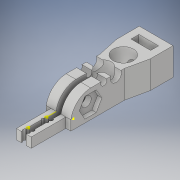
# Autodesk Inventor part: NeuroprobeholdermajigerV3.5SmallerstillStrongerNut
Saved by Autodesk Inventor 2017 (Build 210142000, 142)
## iProperties
Created: 2016-09-01
Part Number: NeuroprobeholdermajigerV3.5SmallerstillStrongerNut
Material: Generic
Document SubType Name: Modeling
Designer: andrew
Density: 1 g/cm^3
Appearance: Default
Author: andrew
Autodesk Inventor part; units mm, degrees
ref_plane "YZ Plane" through (0, 0, 0) normal (1, 0, 0) x (0, 1, 0)
ref_plane "XZ Plane" through (0, 0, 0) normal (0, 1, 0) x (-1, 0, 0)
ref_plane "XY Plane" through (0, 0, 0) normal (0, 0, 1) x (1, 0, 0)
sketch "Sketch1" plane through (0, 0, 0) normal (0, 1, 0) x (-1, 0, 0)
  line L0 (10.16, 7.62) -> (10.16, -36.068)
  line L1 (0, -36.068) -> (0, 3.81) construction
  circle A0 centre (5.08, -25.908) radius 2.9655
  line L2 (10.16, 7.62) -> (6.096, 7.62) construction
  line L3 (3.9775, 7.62) -> (0.0978, 7.62) construction
  line L4 (4.064, 3.81) -> (4.064, -11.0001) construction
  arc A1 (4.064, -14.8101) -> (6.096, -14.812) centre (5.0772, -17.8191) ccw
  line L5 (5.08, -31.75) -> (24.746, -31.75) construction
  line L6 (0, -4.7834) -> (2.794, -4.7834) construction
  line L7 (2.794, -13.6734) -> (0, -13.6734) construction
  line L8 (0, -13.6734) -> (0, -4.7834) construction
  line L9 (4.064, -4.7834) -> (0, -4.7834) construction
  line L10 (5.08, -31.75) -> (9.398, -31.75) construction
  line L11 (10.16, 7.62) -> (6.096, 7.62)
  line L12 (4.064, 7.62) -> (0, 7.62)
  line L13 (0, 0) -> (0, -36.068)
  line L14 (5.08, -36.068) -> (8.255, -36.068) construction
  line L15 (10.16, -36.068) -> (10.16, -39.243)
  line L16 (10.16, -39.243) -> (0, -39.243)
  line L17 (0, -39.243) -> (0, -36.068)
  line L18 (5.0772, -17.8191) -> (26.8769, -17.8191) construction
  arc A2 (4.064, 7.0772) -> (4.064, 5.9038) centre (4.307, 6.4905) ccw
  line L19 (4.064, 7.0772) -> (4.064, 7.62)
  arc A3 (4.064, 5.6778) -> (4.064, 4.0999) centre (4.307, 4.8889) ccw
  line L20 (4.064, -7.1901) -> (4.064, 4.0999)
  line L21 (4.064, 5.6778) -> (4.064, 5.9038)
  line L22 (4.064, 4.0999) -> (4.064, 3.81) construction
  line L23 (4.064, 7.62) -> (4.064, 7.0772) construction
  line L24 (4.064, 5.9038) -> (4.064, 5.6778) construction
  arc A4 (6.0904, 5.9038) -> (6.0904, 7.0772) centre (5.8475, 6.4905) ccw
  arc A5 (6.0904, 4.0999) -> (6.0904, 5.6778) centre (5.8475, 4.8889) ccw
  line L25 (6.096, 7.0749) -> (6.096, 7.62) construction
  line L26 (6.096, 4.1017) -> (6.096, -14.812)
  line L27 (6.096, 7.62) -> (6.096, 7.0749)
  line L28 (6.096, 5.9062) -> (6.096, 5.6761)
  line L29 (6.096, 3.81) -> (6.096, 4.1017) construction
  line L30 (6.096, 5.6761) -> (6.096, 5.9062) construction
  line L31 (0, 0) -> (0, 7.62)
  line L32 (4.064, -7.1901) -> (4.064, -14.8101)
  dimension "d0" = 10.16
  dimension "d1" = 5.9309
  dimension "d2" = 33.528
  dimension "d3" = 6.35
  constraints: 66 end point, 14 point on circle, 10 perpendicular, 6 centre point, 6 horizontal, 4 point on line, 4 vertical, 2 parallel, 1 collinear
  measures "d0" distance of L0.end L1.start
  measures "d1" diameter of A0
  measures "d2" distance from line of L2 A0.centre
  measures "d3" diameter of A1
extrude "Extrusion1" add sketch "Sketch1" along normal blind 4.064
sketch "Sketch3" plane through (0, 0, 7.62) normal (1, 0, 0) x (0, 0, -1)
  line L0 (3.5183, 0) -> (14.9483, 0) construction
  line L1 (3.5183, 0) -> (14.9483, 0) construction
  line L2 (14.9483, 0) -> (14.9483, 3.81) construction
  line L3 (19.5929, 8.2094) -> (17.2434, 4.14) construction
  line L4 (17.2434, 4.14) -> (12.5444, 4.14) construction
  line L5 (12.5444, 4.14) -> (10.1949, 8.2094) construction
  line L6 (10.1949, 8.2094) -> (12.5444, 12.2789) construction
  line L7 (12.5444, 12.2789) -> (17.2434, 12.2789) construction
  line L8 (17.2434, 12.2789) -> (19.5929, 8.2094) construction
  line L9 (14.8939, 4.14) -> (14.8939, 5.4124) construction
  line L10 (10.1949, 8.2094) -> (6.3849, 8.2094) construction
  line L11 (22.4301, 4.064) -> (3.5201, 4.064) construction
  line L12 (10.1949, 8.2094) -> (14.0049, 8.2094) construction
  line L13 (6.3849, 8.2094) -> (6.3849, 0.1438) construction
  line L14 (14.8939, 12.2789) -> (14.8939, 16.4188) construction
  line L15 (14.8939, 16.4188) -> (-4.3508, 16.4188) construction
  line L16 (0, 0) -> (46.863, 0) construction
  line L17 (46.863, 0) -> (46.863, 17.6638) construction
  line L18 (46.863, 0) -> (64.5268, 0) construction
  line L19 (46.863, 0) -> (6.0583, 0)
  line L20 (6.0583, 0) -> (6.0583, 16.4188)
  line L21 (6.0583, 16.4188) -> (46.863, 16.4188)
  line L22 (46.863, 16.4188) -> (46.863, 0)
  line L23 (19.5929, 8.2094) -> (17.2434, 4.14)
  line L24 (17.2434, 4.14) -> (12.5444, 4.14)
  line L25 (12.5444, 4.14) -> (10.1949, 8.2094)
  line L26 (10.1949, 8.2094) -> (12.5444, 12.2789)
  line L27 (12.5444, 12.2789) -> (17.2434, 12.2789)
  line L28 (17.2434, 12.2789) -> (19.5929, 8.2094)
  point P0 (14.8939, 8.2094)
  point P1 (14.8939, 8.2094)
  dimension "d27" = 0
  dimension "d31" = 9.398
  dimension "d35" = 90
  constraints: 54 end point, 4 horizontal, 3 equal length, 3 parallel, 3 perpendicular, 3 vertical, 2 midpoint, 1 coincident, 1 point on line, 26 other
  measures "d27" distance between parallel lines of L0 L1
  measures "d31" distance of L3.start L5.end
  measures "d35" angle of L18 L17
extrude "Extrusion2" add sketch "Sketch3" against normal blind 10.16
sketch "Sketch5" plane through (0, 0, 0) normal (0, -1, 0) x (1, 0, 0)
  arc A0 (-4.0696, 4.0999) -> (-4.0696, 5.6778) centre (-4.3125, 4.8889) ccw
  line L0 (-4.064, 3.81) -> (-4.064, 4.1017) construction
  line L1 (-6.096, 4.0999) -> (-6.096, 3.81) construction
  line L2 (-6.096, 3.81) -> (-6.096, -11.0001) construction
  line L3 (-6.096, -7.1901) -> (-6.096, 4.0999)
  circle A1 centre (-5.08, -25.908) radius 2.9655
  line L4 (-4.064, 4.1017) -> (-4.064, -14.812)
  arc A2 (-6.096, -14.8101) -> (-4.064, -14.812) centre (-5.0828, -17.8191) ccw
  line L5 (-6.096, 5.6778) -> (-6.096, 5.9038)
  line L6 (-6.096, 5.9038) -> (-6.096, 5.6778) construction
  line L7 (-4.064, 5.9062) -> (-4.064, 5.6761)
  line L8 (-4.064, 5.6761) -> (-4.064, 5.9062) construction
  arc A3 (-6.096, 5.6778) -> (-6.096, 4.0999) centre (-5.853, 4.8889) ccw
  arc A4 (-4.0696, 5.9038) -> (-4.0696, 7.0772) centre (-4.3125, 6.4905) ccw
  line L9 (-4.064, 7.0749) -> (-4.064, 7.62) construction
  line L10 (-4.064, 7.62) -> (-4.064, 7.0749)
  line L11 (-6.096, 7.0772) -> (-6.096, 7.62)
  line L12 (-6.096, 7.62) -> (-6.096, 7.0772) construction
  arc A5 (-6.096, 7.0772) -> (-6.096, 5.9038) centre (-5.853, 6.4905) ccw
  line L13 (-5.08, -36.068) -> (-1.905, -36.068) construction
  line L14 (-6.096, -7.1901) -> (-6.096, -14.8101)
  line L15 (-4.064, 7.62) -> (-6.096, 7.62)
  dimension "d41" = 5.9309
  dimension "d43" = 6.35
  constraints: 32 end point, 14 point on circle, 6 centre point, 2 horizontal, 2 point on line, 2 vertical
  measures "d41" diameter of A1
  measures "d43" diameter of A2
extrude "Extrusion4" cut sketch "Sketch5" against normal blind 25.4
sketch "Sketch6" plane through (-10.16, 0, 7.62) normal (-1, 0, 0) x (0, 0, 1)
  line L0 (-17.2434, 4.14) -> (-19.5929, 8.2094) construction
  line L1 (-17.2434, 4.14) -> (-19.5929, 8.2094) construction
  line L2 (-19.5929, 8.2094) -> (-17.2434, 12.2789) construction
  line L3 (-19.5929, 8.2094) -> (-17.2434, 12.2789) construction
  line L4 (-12.5444, 4.14) -> (-17.2434, 4.14) construction
  line L5 (-12.5444, 4.14) -> (-17.2434, 4.14) construction
  line L6 (-10.1949, 8.2094) -> (-12.5444, 4.14) construction
  line L7 (-10.1949, 8.2094) -> (-12.5444, 4.14) construction
  line L8 (-12.5444, 12.2789) -> (-10.1949, 8.2094) construction
  line L9 (-12.5444, 12.2789) -> (-10.1949, 8.2094) construction
  line L10 (-17.2434, 12.2789) -> (-12.5444, 12.2789) construction
  line L11 (-17.2434, 12.2789) -> (-12.5444, 12.2789) construction
  line L12 (-17.7217, 12.9114) -> (-12.2358, 13.0093)
  line L13 (-12.2358, 13.0093) -> (-9.408, 8.3073)
  line L14 (-9.408, 8.3073) -> (-12.0662, 3.5074)
  line L15 (-12.0662, 3.5074) -> (-17.5521, 3.4095)
  line L16 (-17.5521, 3.4095) -> (-20.3798, 8.1115)
  line L17 (-20.3798, 8.1115) -> (-17.7217, 12.9114)
  point P0 (-14.8939, 8.2094)
  constraints: 12 end point, 13 other
extrude "Extrusion5" add sketch "Sketch6" against normal blind 4.064
sketch "Sketch7" plane through (-4.064, 0, 4.0999) normal (-1, 0, 0) x (0, 0, 1)
  line L0 (3.5201, 4.064) -> (-2.5383, 4.064) projected
  line L1 (3.5201, 0) -> (3.5201, 4.064) projected
  line L2 (-43.3429, 0) -> (3.5201, 0) projected
  line L3 (-43.3429, 0) -> (-43.3429, 16.4188) projected
  line L4 (-2.5383, 16.4188) -> (-43.3429, 16.4188) projected
  line L5 (-2.5383, 4.064) -> (-2.5383, 16.4188) projected
  line L6 (-9.0243, 4.14) -> (-6.6748, 8.2094) projected
  line L7 (-6.6748, 8.2094) -> (-9.0243, 12.2789) projected
  line L8 (-9.0243, 12.2789) -> (-13.7233, 12.2789) projected
  line L9 (-13.7233, 12.2789) -> (-16.0728, 8.2094) projected
  line L10 (-16.0728, 8.2094) -> (-13.7233, 4.14) projected
  line L11 (-6.6748, 8.2094) -> (-9.0243, 12.2789) projected
  line L12 (-6.6748, 8.2094) -> (-9.0243, 12.2789) projected
  line L13 (-9.0243, 12.2789) -> (-13.7233, 12.2789) projected
  line L14 (-9.0243, 12.2789) -> (-13.7233, 12.2789) projected
  line L15 (-8.9865, 4.2054) -> (-6.6748, 8.2094) projected
  line L16 (3.5201, 4.064) -> (-2.5383, 4.064) projected
  line L17 (-2.5383, 4.064) -> (0, 4.064) projected
  line L18 (-16.0728, 8.2094) -> (-13.7233, 4.14) projected
  line L19 (-16.0728, 8.2094) -> (-13.7233, 4.14) projected
  line L20 (-13.7233, 12.2789) -> (-16.0728, 8.2094) projected
  line L21 (-13.7233, 12.2789) -> (-16.0728, 8.2094) projected
  line L22 (0, 4.064) -> (1.5779, 4.064) projected
  line L23 (1.5779, 4.064) -> (1.8039, 4.064) projected
  line L24 (1.8039, 4.064) -> (2.9773, 4.064) projected
  line L25 (2.9773, 4.064) -> (3.5201, 4.064) projected
  line L26 (-13.7233, 4.14) -> (-9.0243, 4.14) projected
  point P0 (-4.0999, 0)
  point P1 (-8.7416, 4.064)
  constraints: 1 other
extrude "Extrusion6" add sketch "Sketch7" against normal blind 2.286 contours L26 L10 L9 L8 L7 L6
sketch "Sketch8" plane through (-1.778, 0, 4.0999) normal (1, 0, 0) x (0, 0, -1)
  line L0 (9.0243, 12.2789) -> (13.7233, 12.2789) projected
  line L1 (-3.5201, 4.064) -> (2.5383, 4.064) projected
  circle A0 centre (11.4283, 8.3364) radius 2.0066
  point P0 (4.0999, 0)
  point P1 (8.7416, 4.064)
  point P2 (14.1149, 4.064)
  dimension "d50" = 4.0132
  constraints: 1 centre point
  measures "d50" diameter of A0
extrude "Extrusion7" cut sketch "Sketch8" against normal blind 25.4
fillet "Fillet1" radius 3.175 2 edges at (-6.096, 8.2094, -14.8101) (-4.064, 8.2094, -14.812)
sketch "Sketch9" plane through (0, 16.4188, 1.5617) normal (0, 1, 0) x (1, 0, 0)
  circle A0 centre (-5.08, 27.4697) radius 2.9655 projected
  circle A1 centre (-5.08, 27.4697) radius 4.191
  point P0 (0, 1.5617)
  dimension "d54" = 8.382
  constraints: 1 centre point, 1 coincident
  measures "d54" diameter of A1
extrude "Extrusion8" cut sketch "Sketch9" against normal blind 5.08 contours A0 | A1
sketch "Sketch13" plane through (0, 16.4188, 1.5617) normal (0, 1, 0) x (1, 0, 0)
  circle A0 centre (-5.08, 27.4697) radius 4.191 construction
  arc A1 (-2.9859, 16.9967) -> (-4.064, 14.6126) centre (-0.889, 14.6126) ccw construction
  line L0 (-4.064, 14.6126) -> (-4.064, 0) construction
  line L1 (0, 0) -> (-4.064, 0) construction
  line L2 (0, 0) -> (0, 40.8047) construction
  line L3 (0, 40.8047) -> (-10.16, 40.8047) construction
  line L4 (-10.16, 0) -> (-10.16, 40.8047) construction
  line L5 (-6.096, 0) -> (-10.16, 0) construction
  line L6 (-6.096, 0) -> (-6.096, 14.6078) construction
  arc A2 (-6.096, 14.6078) -> (-7.1769, 16.9942) centre (-9.271, 14.6078) ccw construction
  arc A3 (-2.9859, 16.9967) -> (-7.1769, 16.9942) centre (-5.0828, 19.3807) ccw construction
  line L7 (-5.0846, 23.2787) -> (-5.0846, 34.5411) construction
  line L8 (-5.0846, 23.2787) -> (6.1779, 23.2787) construction
  circle A4 centre (-5.08, 27.4697) radius 4.191 construction
  circle A5 centre (-5.08, 27.4697) radius 4.191 construction
  line L9 (-5.0421, 31.6605) -> (-5.0421, 38.0105) construction
  line L10 (-5.0421, 31.6605) -> (1.3079, 31.6605) construction
  line L11 (-5.0421, 38.0105) -> (15.4873, 38.0105) construction
  line L12 (0, 40.8047) -> (0, -6.0583) projected
  line L13 (0, 38.0105) -> (-11.0208, 38.0105)
  line L14 (-11.0208, 38.0105) -> (-11.0208, 41.2867)
  line L15 (-11.0208, 41.2867) -> (0, 41.2867)
  line L16 (0, 41.2867) -> (0, 38.0105)
  point P0 (0, 1.5617)
  dimension "d63" = 90
  dimension "d64" = 6.35
  dimension "d65" = 90
  dimension "d66" = 90
  constraints: 18 end point, 3 horizontal, 3 parallel, 3 perpendicular, 2 point on line, 1 coincident, 7 other
  measures "d63" angle of L8 L7
  measures "d64" distance of L9.start L9.end
  measures "d65" angle of L10 L9
  measures "d66" angle of L9 L11
extrude "Extrusion11" cut sketch "Sketch13" against normal blind 25.4
sketch "Sketch15" plane through (0, 16.4188, -36.4488) normal (0, 0, -1) x (-1, 0, 0)
  line L0 (10.16, -12.3548) -> (10.16, 0) construction
  line L1 (0, -16.4188) -> (10.16, -16.4188) construction
  line L2 (10.16, -16.4188) -> (10.16, 0) construction
  line L3 (10.16, 0) -> (0, 0) construction
  line L4 (0, 0) -> (0, -16.4188) construction
  line L5 (0, 0) -> (10.16, 0) construction
  line L6 (5.08, 0) -> (5.0828, -16.4188) construction
  line L7 (8.2578, -16.4188) -> (1.9078, -16.4188) construction
  line L8 (10.16, -8.2094) -> (0, -8.2094) construction
  line L9 (10.16, -8.2094) -> (7.62, -12.6088)
  line L10 (7.62, -12.6088) -> (2.54, -12.6088)
  line L11 (2.54, -12.6088) -> (0, -8.2094)
  line L12 (0, -8.2094) -> (2.54, -3.81)
  line L13 (2.54, -3.81) -> (7.62, -3.81)
  line L14 (7.62, -3.81) -> (10.16, -8.2094)
  point P0 (2.9859, -16.4188)
  point P1 (7.1769, -16.4188)
  point P2 (5.08, -8.2094)
  dimension "d76" = 10.16
  constraints: 24 end point, 5 midpoint, 2 parallel, 1 horizontal, 1 perpendicular, 1 point on line, 13 other
  measures "d76" distance of L9.start L11.end
extrude "Extrusion13" cut sketch "Sketch15" against normal blind 1.778
sketch "Sketch16" plane through (0, 16.4188, -34.6708) normal (0, 0, -1) x (-1, 0, 0)
  line L0 (2.54, -3.81) -> (7.62, -3.81) projected
  line L1 (7.62, -12.6088) -> (2.54, -12.6088) projected
  circle A0 centre (5.08, -8.2094) radius 2.0066
  point P0 (0, -16.4188)
  dimension "d79" = 4.0132
  constraints: 1 centre point
  measures "d79" diameter of A0
extrude "Extrusion14" cut sketch "Sketch16" against normal blind 7.62
sketch "Sketch17" plane through (0, 0, 7.62) normal (1, 0, 0) x (0, 0, -1)
  line L0 (10.2086, 16.4188) -> (5.4689, 8.2094) construction
  line L1 (5.4689, 8.2094) -> (10.062, 0.254) construction
  line L2 (24.4278, 8.2094) -> (19.6881, 16.4188) construction
  line L3 (19.6881, 16.4188) -> (10.2086, 16.4188) construction
  line L4 (6.0583, 4.064) -> (6.0583, 16.4188) projected
  arc A0 (14.9483, 21.1494) -> (2.6903, 4.064) centre (14.9483, 8.2094) ccw
  line L5 (6.7389, 8.2094) -> (6.7389, 4.064)
  line L6 (6.7389, 8.2094) -> (10.8523, 8.2094) construction
  line L7 (14.9483, 16.4188) -> (14.9483, 21.1494)
  arc A1 (14.9483, 16.4188) -> (6.7389, 8.2094) centre (14.9483, 8.2094) ccw
  line L8 (2.6903, 4.064) -> (6.7389, 4.064)
  point P0 (7.62, 0)
  dimension "d86" = 270
  constraints: 16 end point, 4 point on circle, 2 centre point, 1 coincident, 1 horizontal, 1 midpoint, 1 vertical
extrude "Extrusion15" cut sketch "Sketch17" against normal blind 12.7
sketch "Sketch19" plane through (0, 0, 0) normal (0, -1, 0) x (1, 0, 0)
  line L0 (0, 7.62) -> (-4.064, 7.62) projected
  line L1 (0, 7.62) -> (-4.064, 7.62)
  line L2 (-4.064, 15.24) -> (-4.064, 14.6972)
  line L3 (-4.064, 13.5238) -> (-4.064, 13.2978)
  line L4 (-4.064, 7.62) -> (0, 7.62)
  arc A0 (-4.064, 11.7199) -> (-4.064, 13.2978) centre (-4.307, 12.5089) ccw
  arc A1 (-4.064, 13.5238) -> (-4.064, 14.6972) centre (-4.307, 14.1105) ccw
  line L5 (0, 15.24) -> (-4.064, 15.24)
  line L6 (-4.064, 11.7199) -> (-4.064, 7.62)
  line L7 (0, 15.24) -> (0, 7.62)
  line L8 (0, 7.62) -> (-4.064, 7.62)
  line L9 (-5.08, 7.62) -> (-5.08, 18.0512)
  line L10 (-10.16, 7.62) -> (-6.096, 7.62)
  line L11 (-10.16, 7.62) -> (-6.096, 7.62)
  line L12 (-6.096, 15.24) -> (-6.096, 14.6972)
  line L13 (-6.096, 13.5238) -> (-6.096, 13.2978)
  line L14 (-6.096, 7.62) -> (-10.16, 7.62)
  arc A2 (-6.096, 13.2978) -> (-6.096, 11.7199) centre (-5.853, 12.5089) ccw
  arc A3 (-6.096, 14.6972) -> (-6.096, 13.5238) centre (-5.853, 14.1105) ccw
  line L15 (-10.16, 15.24) -> (-6.096, 15.24)
  line L16 (-6.096, 11.7199) -> (-6.096, 7.62)
  line L17 (-10.16, 15.24) -> (-10.16, 7.62)
  line L18 (-10.16, 7.62) -> (-6.096, 7.62)
  point P0 (-6.096, 7.62)
  constraints: 36 end point, 12 symmetric about line, 8 point on circle, 4 centre point, 3 collinear, 2 vertical, 1 perpendicular, 2 other
extrude "Extrusion16" add sketch "Sketch19" against normal blind 4.064
sketch "Sketch20" plane through (0, 4.064, 0) normal (0, 1, 0) x (1, 0, 0)
  line L0 (-4.064, -15.24) -> (0, -15.24) construction
  line L1 (-4.064, -15.24) -> (0, -15.24) construction
  line L2 (-2.032, -15.24) -> (-2.032, -0.8811) construction
  line L3 (0, -0.8811) -> (-4.064, -0.8811) construction
  line L4 (-4.064, -7.0772) -> (-4.064, -11.7199) construction
  line L5 (-4.064, -8.8304) -> (-6.1163, -8.8304) construction
  line L6 (-5.0902, -8.8304) -> (-5.0902, -11.9268) construction
  line L7 (-2.032, -15.24) -> (0, -15.24)
  line L8 (0, -15.24) -> (0, -0.8811)
  line L9 (0, -0.8811) -> (-2.032, -0.8811)
  line L10 (-2.032, -0.8811) -> (-2.032, -15.24)
  line L11 (-6.1163, -15.24) -> (-10.1803, -15.24) construction
  line L12 (-6.1163, -15.24) -> (-10.1803, -15.24) construction
  line L13 (-8.1483, -15.24) -> (-8.1483, -0.8811) construction
  line L14 (-10.1803, -0.8811) -> (-6.1163, -0.8811) construction
  line L15 (-6.1163, -7.0772) -> (-6.1163, -11.7199) construction
  line L16 (-6.1163, -8.8304) -> (-4.064, -8.8304) construction
  line L17 (-8.1483, -15.24) -> (-10.1803, -15.24)
  line L18 (-10.1803, -15.24) -> (-10.1803, -0.8811)
  line L19 (-10.1803, -0.8811) -> (-8.1483, -0.8811)
  line L20 (-8.1483, -0.8811) -> (-8.1483, -15.24)
  point P0 (0, 0)
  point P1 (-10.1803, 0)
  constraints: 36 end point, 13 symmetric about line, 3 horizontal, 3 midpoint, 2 parallel, 2 point on line, 1 perpendicular, 1 vertical
extrude "Extrusion17" cut sketch "Sketch20" against normal blind 4.064
sketch "Sketch22" plane through (0, 0, 0) normal (0, -1, 0) x (1, 0, 0)
  line L0 (-7.62, -34.6708) -> (-2.54, -34.6708) construction
  line L1 (-12.065, -34.6708) -> (-12.065, -39.4968) construction
  line L2 (-12.065, -39.4968) -> (4.1708, -39.4968) construction
  line L3 (-12.065, -34.6708) -> (-12.065, -39.4968)
  line L4 (-12.065, -39.4968) -> (1.905, -39.4968)
  line L5 (1.905, -39.4968) -> (1.905, -34.6708)
  line L6 (-12.065, -34.6708) -> (-12.065, -33.1595)
  line L7 (1.905, -34.6708) -> (1.905, -33.1595)
  line L8 (0, -36.4488) -> (0, 0.8811) projected
  line L9 (-10.16, 0.8811) -> (-10.16, -36.4488) projected
  line L10 (-10.16, -33.1595) -> (-10.16, -36.4488)
  line L11 (-10.16, -36.4488) -> (0, -36.4488)
  line L12 (0, -36.4488) -> (0, -33.1595)
  line L13 (1.905, -33.1595) -> (1.905, -29.3495)
  line L14 (-12.065, -33.1595) -> (-12.065, -29.3495)
  line L15 (-12.065, -29.3495) -> (-10.16, -29.3495)
  line L16 (1.905, -29.3495) -> (0, -29.3495)
  point P0 (0, 0)
  dimension "d94" = 13.97
  dimension "d95" = 4.826
  dimension "d102" = 1.5113
  dimension "d105" = 3.81
  constraints: 28 end point, 5 vertical, 3 perpendicular, 3 point on line, 2 parallel
  measures "d94" distance of L1.start L5.end
  measures "d95" distance of L1.start L1.end
  measures "d102" distance of L3.start L6.end
  measures "d105" distance of L7.end L13.end
sketch "Sketch24" plane through (-10.16, 16.4188, -36.4488) normal (0, 1, 0) x (1, 0, 0)
  line L0 (10.16, 0) -> (0, 0)
  line L1 (0, 0) -> (0, -1.778)
  line L2 (0, -1.778) -> (10.16, -1.778)
  line L3 (10.16, -1.778) -> (10.16, 0)
  point P0 (10.16, -36.4488)
  constraints: 8 end point, 2 parallel, 1 horizontal, 1 perpendicular
extrude "Extrusion20" cut sketch "Sketch24" against normal blind 8.2042
sketch "Sketch25" plane through (0, 16.4188, -34.6708) normal (0, 0, -1) x (-1, 0, 0)
  line L0 (0, -8.2094) -> (0.003, -8.2042) projected
  line L1 (2.54, -12.6088) -> (0, -8.2094) projected
  line L2 (7.62, -12.6088) -> (2.54, -12.6088) projected
  line L3 (10.16, -8.2094) -> (7.62, -12.6088) projected
  line L4 (10.157, -8.2042) -> (10.16, -8.2094) projected
  line L5 (10.157, -8.2042) -> (10.16, -8.2042) projected
  line L6 (10.16, 0) -> (10.16, -8.2042) projected
  line L7 (0, 0) -> (10.16, 0) projected
  line L8 (0, -8.2042) -> (0, 0) projected
  line L9 (0, -8.2042) -> (0.003, -8.2042) projected
  circle A0 centre (5.08, -8.2094) radius 2.0066 projected
  point P0 (0, -16.4188)
  dimension "d127" = 10.16
  measures "d127" distance between parallel lines of L8 L6
extrude "Extrusion21" cut sketch "Sketch25" against normal blind 1.5113
extrude "Extrusion22" add sketch "Sketch22" against normal blind 16.4084
fillet "Fillet2" radius 1.27 4 edges at (1.905, 8.2042, -29.3495) (0, 8.2042, -29.3495) (-12.065, 8.2042, -29.3495) (-10.16, 8.2042, -29.3495)
sketch "Sketch26" plane through (1.905, 0, -39.4968) normal (0, 0, -1) x (-1, 0, 0)
  circle A0 centre (6.985, 8.2094) radius 2.0066 projected
  point P0 (1.905, 0)
  constraints: 1 other
extrude "Extrusion23" cut sketch "Sketch26" against normal blind 15.24
sketch "Sketch27" plane through (1.905, 0, -39.4968) normal (1, 0, 0) x (0, 0, -1)
  line L0 (-34.5724, 12.2789) -> (-29.8734, 12.2789) projected
  line L1 (-32.1685, 14.1088) -> (6.9816, 14.1088)
  line L2 (6.9816, 14.1088) -> (6.9816, 23.872)
  line L3 (6.9816, 23.872) -> (-40.3779, 23.872)
  line L4 (-40.3779, 23.872) -> (-40.3779, 6.7927)
  line L5 (-46.574, 4.064) -> (-45.4007, 4.064) projected
  line L6 (-40.3779, 4.064) -> (-40.3779, 8.2094) projected
  line L7 (-40.3779, 4.064) -> (-40.3779, 4.064)
  circle A0 centre (-32.1685, 8.2094) radius 5.8994 construction
  line L8 (-40.3779, 4.064) -> (-43.5967, 4.064) projected
  arc A1 (-32.1685, 14.1088) -> (-40.3779, 6.7927) centre (-31.7973, 5.4283) ccw
  point P0 (-39.4968, 0)
  dimension "d110" = 90
  constraints: 10 end point, 3 perpendicular, 2 centre point, 2 point on circle, 2 point on line, 1 tangent
  measures "d110" angle of L4 L3
extrude "Extrusion24" cut sketch "Sketch27" against normal blind 25.4
sketch "Sketch28" plane through (0, 4.064, 0) normal (0, 1, 0) x (1, 0, 0)
  line L0 (-2.032, -15.24) -> (-2.032, -0.8811) projected
  line L1 (-2.032, -0.8811) -> (-4.064, -0.8811) projected
  line L2 (-4.064, -0.8811) -> (-4.064, -4.0999) projected
  arc A0 (-4.064, -5.6778) -> (-4.064, -4.0999) centre (-4.307, -4.8889) ccw projected
  line L3 (-4.064, -5.6778) -> (-4.064, -5.9038) projected
  arc A1 (-4.064, -7.0772) -> (-4.064, -5.9038) centre (-4.307, -6.4905) ccw projected
  line L4 (-4.064, -7.0772) -> (-4.064, -11.7199) projected
  arc A2 (-4.064, -13.2978) -> (-4.064, -11.7199) centre (-4.307, -12.5089) ccw projected
  line L5 (-4.064, -13.2978) -> (-4.064, -13.5238) projected
  arc A3 (-4.064, -14.6972) -> (-4.064, -13.5238) centre (-4.307, -14.1105) ccw projected
  line L6 (-4.064, -14.6972) -> (-4.064, -15.24) projected
  line L7 (-4.064, -15.24) -> (-2.032, -15.24) projected
  line L8 (-8.1483, -0.8811) -> (-8.1483, -15.24) projected
  line L9 (-8.1483, -15.24) -> (-6.096, -15.24) projected
  line L10 (-6.096, -15.24) -> (-6.096, -14.6972) projected
  arc A4 (-6.096, -13.5238) -> (-6.096, -14.6972) centre (-5.853, -14.1105) ccw projected
  line L11 (-6.096, -13.5238) -> (-6.096, -13.2978) projected
  arc A5 (-6.096, -11.7199) -> (-6.096, -13.2978) centre (-5.853, -12.5089) ccw projected
  line L12 (-6.096, -11.7199) -> (-6.096, -7.0772) projected
  arc A6 (-6.096, -5.9038) -> (-6.096, -7.0772) centre (-5.853, -6.4905) ccw projected
  line L13 (-6.096, -5.9038) -> (-6.096, -5.6778) projected
  arc A7 (-6.096, -4.0999) -> (-6.096, -5.6778) centre (-5.853, -4.8889) ccw projected
  line L14 (-6.096, -4.0999) -> (-6.096, -0.8811) projected
  line L15 (-6.096, -0.8811) -> (-8.1483, -0.8811) projected
  point P0 (0, 0)
extrude "Extrusion25" add sketch "Sketch28" along normal blind 2.7178 and the other way blind 1.3462
sketch "Sketch29" plane through (0, 0, 0) normal (0, -1, 0) x (1, 0, 0)
  line L0 (4.0115, -40.7723) -> (-15.4869, -40.7723)
  line L1 (-15.4869, -40.7723) -> (-15.4869, 20.2217)
  line L2 (-15.4869, 20.2217) -> (4.0115, 20.2217)
  line L3 (4.0115, 20.2217) -> (4.0115, -40.7723)
  point P0 (0, 0)
  constraints: 8 end point, 2 parallel, 1 horizontal, 1 perpendicular
extrude "Extrusion26" cut sketch "Sketch29" against normal blind 2.7178
sketch "Sketch30" plane through (0, 14.1088, -7.3283) normal (1, 0, 0) x (0, 0, -1)
  line L0 (0, 0) -> (11.002, 0) construction
  circle A0 centre (5.4184, -0.6667) radius 1.27
  line L1 (-3.81, 0) -> (35.433, 0) construction
  line L2 (3.0307, 0) -> (3.0307, 0.508)
  line L3 (3.0307, 0) -> (3.5387, 0) construction
  line L4 (3.5143, -0.5477) -> (3.5143, -0.7064)
  line L5 (3.5143, -0.5477) -> (3.6731, -0.5477) construction
  line L6 (19.1326, 0) -> (25.0635, 0) construction
  line L7 (25.0635, -19.05) -> (25.0635, 0) construction
  circle A1 centre (10.4392, -0.9712) radius 2.286
  point P0 (-7.3283, -14.1088)
  point P1 (32.258, 0)
  point P2 (28.8734, 0)
  point P3 (28.8734, 9.525)
  point P4 (0, 0)
  dimension "d119" = 2.54
  dimension "d120" = 0.508
  dimension "d121" = 90
  dimension "d122" = 0.1588
  dimension "d123" = 90
  dimension "d124" = 4.572
  constraints: 14 end point, 3 perpendicular, 2 centre point, 2 horizontal, 1 point on line, 1 vertical, 3 other
  measures "d119" diameter of A0
  measures "d120" distance of L2.start L2.end
  measures "d121" angle of L3 L2
  measures "d122" distance of L4.start L4.end
  measures "d123" angle of L4 L5
  measures "d124" diameter of A1
extrude "Extrusion27" cut sketch "Sketch30" against normal blind 25.4
sketch "Sketch31" plane through (0, 6.7818, 0) normal (0, 1, 0) x (1, 0, 0)
  arc A0 (-6.096, -4.0999) -> (-6.096, -5.6778) centre (-5.853, -4.8889) ccw projected
  arc A1 (-6.096, -11.7199) -> (-6.096, -13.2978) centre (-5.853, -12.5089) ccw projected
  line L0 (-6.096, -4.0999) -> (-6.096, -0.8811) projected
  point P0 (0, 0)
sketch "Sketch32" plane through (1.905, 14.1088, -30.6195) normal (0, 1, 0) x (1, 0, 0)
  line L0 (-12.065, 5.8293) -> (-12.065, 2.54) projected
  line L1 (-1.905, 2.54) -> (-1.905, 5.8293) projected
  line L2 (-12.065, 5.8293) -> (-9.525, 5.8293) projected
  line L3 (-12.065, 2.54) -> (-11.049, 2.54)
  line L4 (-11.049, 2.54) -> (-11.049, 5.8293)
  line L5 (-11.049, 5.8293) -> (-12.065, 5.8293)
  line L6 (-12.065, 5.8293) -> (-12.065, 2.54)
  line L7 (-12.065, 2.54) -> (-1.905, 2.54) projected
  line L8 (-1.905, 5.8293) -> (-2.921, 5.8293)
  line L9 (-2.921, 5.8293) -> (-2.921, 2.54)
  line L10 (-2.921, 2.54) -> (-1.905, 2.54)
  line L11 (-1.905, 2.54) -> (-1.905, 5.8293)
  point P0 (-1.905, -30.6195)
  dimension "d128" = 1.016
  dimension "d129" = 1.016
  constraints: 16 end point, 4 parallel, 2 horizontal, 2 perpendicular, 2 point on line
  measures "d128" distance of L5.end L4.end
  measures "d129" distance of L10.end L9.end
extrude "Extrusion28" add sketch "Sketch32" against normal blind 10.16
sketch "Sketch33" plane through (-5.08, 11.3388, -25.908) normal (0, 1, 0) x (1, 0, 0)
  circle A0 centre (0, 0) radius 4.191 projected
  point P0 (5.08, -25.908)
extrude "Extrusion29" cut sketch "Sketch33" against normal blind 25.4
sketch "Sketch34" plane through (1.905, 14.1088, -30.6195) normal (0, 1, 0) x (1, 0, 0)
  circle A0 centre (-6.985, -4.7115) radius 4.191 projected
  line L0 (-2.921, 5.8293) -> (-2.921, 2.54) projected
  line L1 (-11.049, 2.54) -> (-2.921, 2.54) projected
  line L2 (-11.049, 2.54) -> (-11.049, 5.8293) projected
  line L3 (-2.921, 5.8293) -> (-11.049, 5.8293) projected
  line L4 (-4.5365, -10.7825) -> (-1.905, -10.7825) projected
  line L5 (-1.905, -2.4593) -> (-1.905, -10.7825) projected
  arc A1 (-0.9525, -1.2297) -> (-1.905, -2.4593) centre (-0.635, -2.4593) ccw projected
  arc A2 (-0.9525, -1.2297) -> (0, 0) centre (-1.27, 0) ccw projected
  line L6 (0, 8.8773) -> (0, 0) projected
  line L7 (-13.97, 8.8773) -> (0, 8.8773) projected
  line L8 (-13.97, 0) -> (-13.97, 8.8773) projected
  arc A3 (-13.97, 0) -> (-13.0175, -1.2297) centre (-12.7, 0) ccw projected
  arc A4 (-12.065, -2.4593) -> (-13.0175, -1.2297) centre (-13.335, -2.4593) ccw projected
  line L9 (-12.065, -10.7825) -> (-12.065, -2.4593) projected
  line L10 (-12.065, -10.7825) -> (-9.439, -10.7825) projected
  arc A5 (-4.5365, -10.7825) -> (-9.439, -10.7825) centre (-6.9878, -12.8005) ccw projected
  circle A6 centre (-6.985, -4.7115) radius 4.191 projected
  line L11 (-6.9964, -8.9025) -> (-6.9878, -9.6255)
  line L12 (-6.9921, -9.264) -> (-12.065, -9.264)
  arc A7 (-13.97, 0) -> (-13.0175, -1.2297) centre (-12.7, 0) ccw projected
  line L13 (-12.065, -9.264) -> (-13.97, -0.5205)
  line L14 (-13.97, -0.5205) -> (-13.97, 0)
  line L15 (-6.9921, -9.264) -> (-1.905, -9.264)
  line L16 (-1.905, -9.264) -> (0, -0.5205)
  line L17 (0, -0.5205) -> (0, 0)
  line L18 (-1.905, -2.4593) -> (-1.905, -10.7825) projected
  line L19 (-1.905, -9.264) -> (-1.905, 0)
  line L20 (-1.905, 0) -> (0, 0)
  line L21 (-12.065, -9.264) -> (-12.065, 0)
  line L22 (-13.97, 0) -> (-12.065, 0)
  point P0 (-1.905, -30.6195)
  constraints: 22 end point, 4 point on line, 3 perpendicular, 3 tangent, 2 vertical, 1 horizontal, 1 midpoint, 1 parallel, 1 point on circle, 4 other
extrude "Extrusion30" add sketch "Sketch34" against normal blind 25.4 contours L5 A1 A2 L17 L16 | L13 L14 A3 A4 L9
sketch "Sketch35" plane through (0, 2.7178, 0.8811) normal (1, 0, 0) x (0, 0, -1)
  line L0 (40.3779, 0) -> (40.3779, 11.391) projected
  line L1 (40.3779, 0) -> (17.4781, 0)
  line L2 (17.4781, 0) -> (17.4781, -17.3176)
  line L3 (17.4781, -17.3176) -> (40.3779, -17.3176)
  line L4 (40.3779, -17.3176) -> (40.3779, 0)
  point P0 (0.8811, -2.7178)
  constraints: 8 end point, 2 parallel, 1 horizontal, 1 perpendicular
extrude "Extrusion31" cut sketch "Sketch35" along normal blind 25.4 and the other way blind 12.7
sketch "Sketch36" plane through (-7.62, 3.81, -33.1595) normal (0, 1, 0) x (1, 0, 0)
  line L0 (0, 3.2893) -> (5.08, 3.2893) construction
  line L1 (0, 3.2893) -> (0, 0) construction
  line L2 (0, 0) -> (5.08, 0) construction
  line L3 (5.08, 3.2893) -> (5.08, 0) construction
  line L4 (0, 1.6447) -> (5.08, 1.6446) construction
  line L5 (2.54, 1.6446) -> (2.54, 3.2893) construction
  circle A0 centre (2.54, 1.6446) radius 0.9525
  point P0 (7.62, -33.1595)
  dimension "d140" = 1.905
  constraints: 4 end point, 4 midpoint, 1 centre point, 1 coincident
  measures "d140" diameter of A0
extrude "Extrusion32" cut sketch "Sketch36" against normal blind 25.4
body "Solid1"
